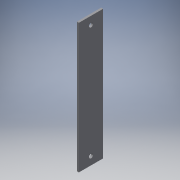
# Autodesk Inventor part: 15102898-16-P-0405
Saved by Autodesk Inventor 2017 (Build 210142000, 142)
## iProperties
Created: 2016-10-08
Part Number: 15102898-16-P-0405
Material: Polycarbonate, Clear
Document SubType Name: Modeling
Designer: gus
Density: 1.2 g/cm^3
Appearance: Polycarbonate - Clear
Author: gus
Autodesk Inventor part; units mm, degrees
ref_plane "YZ Plane" through (0, 0, 0) normal (1, 0, 0) x (0, 1, 0)
ref_plane "XZ Plane" through (0, 0, 0) normal (0, 1, 0) x (-1, 0, 0)
ref_plane "XY Plane" through (0, 0, 0) normal (0, 0, 1) x (1, 0, 0)
sketch "Sketch1" plane through (0, 0, 0) normal (1, 0, 0) x (0, 1, 0)
  line L0 (0, 0) -> (215.9, 0)
  line L1 (215.9, 0) -> (215.9, 38.1)
  line L2 (215.9, 38.1) -> (0, 38.1)
  line L3 (0, 38.1) -> (0, 0)
  circle A0 centre (12.7, 19.05) radius 3.175
  circle A1 centre (203.2, 19.05) radius 3.175
  dimension "d1" = 38.1
  dimension "d2" = 19.05
  dimension "d3" = 12.7
  dimension "d4" = 12.7
  dimension "d5" = 19.05
  dimension "d6" = 6.35
  dimension "d9" = 190.5
  constraints: 8 end point, 2 centre point, 2 parallel, 1 equal radius, 1 horizontal, 1 perpendicular
  measures "d1" distance of L1.end L0.end
  measures "d2" distance from line of L2 A0.centre
  measures "d3" distance from line of L3 A0.centre
  measures "d4" distance from line of L1 A1.centre
  measures "d5" distance from line of L2 A1.centre
  measures "d6" diameter of A0
  measures "d9" distance of A1.centre A0.centre
extrude "Extrusion1" add sketch "Sketch1" along normal blind 3.175
body "Solid1"
